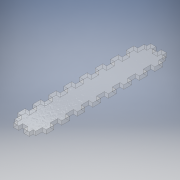
# Autodesk Inventor part: case_back
Saved by Autodesk Inventor 2019 (Build 230136000, 136)
## iProperties
Created: 2019-02-02
Part Number: case_back
Material: Acrylic, Clear
Document SubType Name: Modeling
Designer: suchanek
Density: 1.19 g/cm^3
Appearance: Transparent - Clear
Author: suchanek
Autodesk Inventor part; units mm, degrees
ref_plane "YZ Plane" through (0, 0, 0) normal (1, 0, 0) x (0, 1, 0)
ref_plane "XZ Plane" through (0, 0, 0) normal (0, 1, 0) x (-1, 0, 0)
ref_plane "XY Plane" through (0, 0, 0) normal (0, 0, 1) x (1, 0, 0)
sketch "Sketch1" plane through (0, 0, 0) normal (0, 1, 0) x (-1, 0, 0)
  line L0 (-16.25, 100) -> (16.25, 100)
  line L1 (16.25, 100) -> (16.25, -100)
  line L2 (16.25, -100) -> (-16.25, -100)
  line L3 (-16.25, -100) -> (-16.25, 100)
  line L4 (-16.25, 100) -> (16.25, -100) construction
  line L5 (16.25, 100) -> (-16.25, -100) construction
  line L6 (-16.25, 90) -> (-22.25, 90)
  line L7 (-22.25, 90) -> (-22.25, 78)
  line L8 (-22.25, 78) -> (-16.25, 78)
  line L9 (-16.25, 78) -> (-16.25, 90)
  line L10 (-22.25, 66) -> (-16.25, 66)
  line L11 (-16.25, 66) -> (-16.25, 54)
  line L12 (-16.25, 54) -> (-22.25, 54)
  line L13 (-22.25, 54) -> (-22.25, 66)
  line L14 (-16.25, 42) -> (-22.25, 42)
  line L15 (-22.25, 42) -> (-22.25, 30)
  line L16 (-22.25, 30) -> (-16.25, 30)
  line L17 (-16.25, 30) -> (-16.25, 42)
  line L18 (-16.25, 18) -> (-22.25, 18)
  line L19 (-22.25, 18) -> (-22.25, 6)
  line L20 (-22.25, 6) -> (-16.25, 6)
  line L21 (-16.25, 6) -> (-16.25, 18)
  line L22 (0, 0) -> (-5.6352, 0)
  line L23 (-5.6352, 0) -> (0, 0)
  line L24 (0, 0) -> (0, 8.7024)
  line L25 (-16.25, 100) -> (16.25, -100) construction
  line L26 (16.25, 90) -> (22.25, 90)
  line L27 (22.25, 90) -> (22.25, 78)
  line L28 (22.25, 78) -> (16.25, 78)
  line L29 (16.25, 78) -> (16.25, 90)
  line L30 (22.25, 66) -> (16.25, 66)
  line L31 (16.25, 66) -> (16.25, 54)
  line L32 (16.25, 54) -> (22.25, 54)
  line L33 (22.25, 54) -> (22.25, 66)
  line L34 (16.25, 42) -> (22.25, 42)
  line L35 (22.25, 42) -> (22.25, 30)
  line L36 (22.25, 30) -> (16.25, 30)
  line L37 (16.25, 30) -> (16.25, 42)
  line L38 (16.25, 18) -> (22.25, 18)
  line L39 (22.25, 18) -> (22.25, 6)
  line L40 (22.25, 6) -> (16.25, 6)
  line L41 (16.25, 6) -> (16.25, 18)
  line L42 (-16.25, -90) -> (-22.25, -90)
  line L43 (-22.25, -90) -> (-22.25, -78)
  line L44 (-22.25, -78) -> (-16.25, -78)
  line L45 (-16.25, -78) -> (-16.25, -90)
  line L46 (-22.25, -66) -> (-16.25, -66)
  line L47 (-16.25, -66) -> (-16.25, -54)
  line L48 (-16.25, -54) -> (-22.25, -54)
  line L49 (-22.25, -54) -> (-22.25, -66)
  line L50 (-16.25, -42) -> (-22.25, -42)
  line L51 (-22.25, -42) -> (-22.25, -30)
  line L52 (-22.25, -30) -> (-16.25, -30)
  line L53 (-16.25, -30) -> (-16.25, -42)
  line L54 (-16.25, -18) -> (-22.25, -18)
  line L55 (-22.25, -18) -> (-22.25, -6)
  line L56 (-22.25, -6) -> (-16.25, -6)
  line L57 (-16.25, -6) -> (-16.25, -18)
  line L58 (22.25, -42) -> (22.25, -30)
  line L59 (16.25, -30) -> (16.25, -42)
  line L60 (16.25, -6) -> (16.25, -18)
  line L61 (22.25, -6) -> (16.25, -6)
  line L62 (22.25, -18) -> (22.25, -6)
  line L63 (16.25, -18) -> (22.25, -18)
  line L64 (22.25, -30) -> (16.25, -30)
  line L65 (16.25, -90) -> (22.25, -90)
  line L66 (22.25, -90) -> (22.25, -78)
  line L67 (22.25, -78) -> (16.25, -78)
  line L68 (16.25, -78) -> (16.25, -90)
  line L69 (16.25, -42) -> (22.25, -42)
  line L70 (16.25, -54) -> (22.25, -54)
  line L71 (16.25, -66) -> (16.25, -54)
  line L72 (22.25, -66) -> (16.25, -66)
  line L73 (22.25, -54) -> (22.25, -66)
  line L74 (12.25, 100) -> (4, 100)
  line L75 (4, 100) -> (4, 106)
  line L76 (4, 106) -> (12.25, 106)
  line L77 (12.25, 106) -> (12.25, 100)
  line L78 (-12.25, 100) -> (-4, 100)
  line L79 (-4, 100) -> (-4, 106)
  line L80 (-4, 106) -> (-12.25, 106)
  line L81 (-12.25, 106) -> (-12.25, 100)
  line L82 (12.25, -100) -> (4, -100)
  line L83 (4, -100) -> (4, -106)
  line L84 (4, -106) -> (12.25, -106)
  line L85 (12.25, -106) -> (12.25, -100)
  line L86 (-12.25, -100) -> (-4, -100)
  line L87 (-4, -100) -> (-4, -106)
  line L88 (-4, -106) -> (-12.25, -106)
  line L89 (-12.25, -106) -> (-12.25, -100)
  point P0 (0, -8.7024)
  dimension "d0" = 32.5
  dimension "d1" = 200
  dimension "d2" = 6
  dimension "d3" = 6
  dimension "d4" = 12
  dimension "d5" = 12
  dimension "d6" = 12
  dimension "d7" = 12
  dimension "d8" = 12
  dimension "d9" = 12
  dimension "d10" = 12
  dimension "d17" = 6
  dimension "d18" = 4
  dimension "d19" = 4
  constraints: 180 end point, 61 symmetric about line, 17 point on line, 13 equal length, 7 horizontal, 6 perpendicular, 2 midpoint, 1 vertical
  measures "d0" distance of L1.end L2.end
  measures "d1" distance of L0.end L1.end
  measures "d2" distance of L19.end L20.end
  measures "d3" distance from line of L22.start L20
  measures "d4" distance of L18.end L19.end
  measures "d5" distance between parallel lines of L18 L16
  measures "d6" distance of L14.end L15.end
  measures "d7" distance between parallel lines of L12 L14
  measures "d8" distance of L12.end L10.start
  measures "d9" distance between parallel lines of L10 L8
  measures "d10" distance of L6.end L7.end
  measures "d17" distance of L74.end L75.end
  measures "d18" distance between parallel lines of L1 L77
  measures "d19" distance between parallel lines of L24 L75
extrude "Extrusion1" add sketch "Sketch1" along normal blind 6
body "Solid1"
